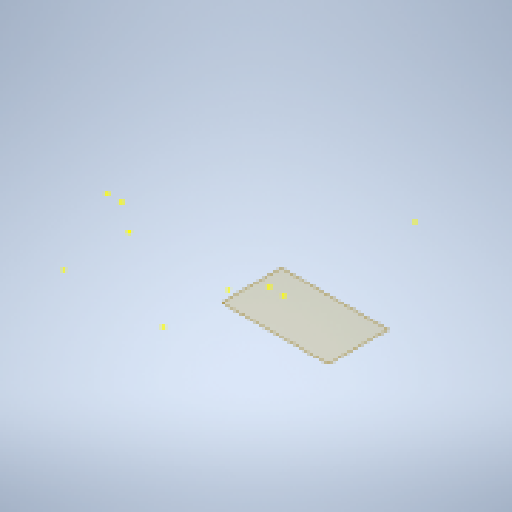
# Autodesk Inventor part: OCOTPUS_BOX_BACKING
Saved by Autodesk Inventor 2025.2 (Build 292293000, 293)
## iProperties
Created: 2026-03-26
Part Number: OCOTPUS_BOX_BACKING
Material: Generic
Document SubType Name: Sheet Metal
Designer: composite
Density: 1 g/cm^3
Sheet Metal Rule: Default_mm
Appearance: Default
Author: composite
Autodesk Inventor part; units mm, degrees
ref_plane "YZ Plane" through (0, 0, 0) normal (1, 0, 0) x (0, 1, 0)
ref_plane "XZ Plane" through (0, 0, 0) normal (0, 1, 0) x (-1, 0, 0)
ref_plane "XY Plane" through (0, 0, 0) normal (0, 0, 1) x (1, 0, 0)
ref_plane "Work Plane1" through (45.6354, 347.161, 237.8796) normal (0, 1, 0) x (-1, 0, 0)
sketch "Sketch1" plane through (45.6354, 347.161, 237.8796) normal (0, 1, 0) x (-1, 0, 0)
  circle A0 centre (74.35, -12.65) radius 2.75 projected
  circle A1 centre (49.35, -12.65) radius 2.75 projected
  circle A2 centre (355.85, -12.65) radius 2.75 projected
  circle A3 centre (330.85, -12.65) radius 2.75 projected
  circle A4 centre (278.85, 26.85) radius 2 projected
  circle A5 centre (278.85, 139.85) radius 2 projected
  circle A6 centre (105.85, 139.85) radius 2 projected
  circle A7 centre (105.85, 26.85) radius 2 projected
  line L0 (102.35, 141.35) -> (102.35, 25.35) projected
  circle A8 centre (105.85, 26.85) radius 3 projected
  circle A9 centre (278.85, 139.85) radius 3 projected
  circle A10 centre (117.35, 38.35) radius 1.75 projected
  circle A11 centre (267.35, 128.35) radius 1.75 projected
  circle A12 centre (267.35, 38.35) radius 1.75 projected
  circle A13 centre (117.35, 128.35) radius 1.75 projected
  arc A14 (280.35, 23.35) -> (282.35, 25.35) centre (280.35, 25.35) ccw projected
  line L1 (104.35, 23.35) -> (280.35, 23.35) projected
  arc A15 (102.35, 25.35) -> (104.35, 23.35) centre (104.35, 25.35) ccw projected
  line L2 (102.35, 141.35) -> (102.35, 25.35) projected
  arc A16 (104.35, 143.35) -> (102.35, 141.35) centre (104.35, 141.35) ccw projected
  line L3 (280.35, 143.35) -> (104.35, 143.35) projected
  arc A17 (282.35, 141.35) -> (280.35, 143.35) centre (280.35, 141.35) ccw projected
  line L4 (282.35, 25.35) -> (282.35, 141.35) projected
  circle A18 centre (105.85, 139.85) radius 3 projected
  circle A19 centre (278.85, 26.85) radius 3 projected
  line L5 (-3.9627, -32.65) -> (79.35, -32.65) projected
  line L6 (409.1627, -32.65) -> (325.85, -32.65) projected
  point P0 (45.6354, -237.8796)
sketch "Sketch2" plane through (45.6354, 347.161, 237.8796) normal (0, 1, 0) x (-1, 0, 0)
  arc A0 (104.35, 143.35) -> (102.35, 141.35) centre (104.35, 141.35) ccw
  line L0 (280.35, 143.35) -> (104.35, 143.35)
  arc A1 (282.35, 141.35) -> (280.35, 143.35) centre (280.35, 141.35) ccw
  circle A2 centre (278.85, 139.85) radius 2
  circle A3 centre (105.85, 139.85) radius 2
  circle A4 centre (105.85, 26.85) radius 2
  circle A5 centre (278.85, 26.85) radius 2
  line L1 (104.35, 23.35) -> (280.35, 23.35)
  circle A6 centre (330.85, -12.65) radius 2.75
  circle A7 centre (355.85, -12.65) radius 2.75
  circle A8 centre (49.35, -12.65) radius 2.75
  circle A9 centre (74.35, -12.65) radius 2.75
  line L2 (-3.9627, -32.65) -> (79.35, -32.65)
  line L3 (409.1627, -32.65) -> (325.85, -32.65)
  circle A10 centre (74.35, -12.65) radius 3.25
  circle A11 centre (49.35, -12.65) radius 3.25
  circle A12 centre (330.85, -12.65) radius 3.25
  circle A13 centre (355.85, -12.65) radius 3.25
  line L4 (79.35, -32.65) -> (115.85, 23.35)
  line L5 (115.85, 23.35) -> (268.85, 23.35)
  line L6 (268.85, 23.35) -> (325.85, -32.65)
  line L7 (370.85, -32.65) -> (370.85, 7.35)
  line L8 (370.85, 7.35) -> (282.35, 68.35)
  line L9 (282.35, 68.35) -> (282.35, 141.35)
  line L10 (34.35, -32.65) -> (34.35, 7.35)
  line L11 (34.35, 7.35) -> (102.35, 83.35)
  line L12 (102.35, 141.35) -> (102.35, 83.35)
  point P0 (45.6354, -237.8796)
  dimension "d0" = 0.5
  dimension "d1" = 0.5
  dimension "d2" = 0.5
  dimension "d3" = 0.5
  dimension "d4" = 45
  dimension "d5" = 45
  dimension "d6" = 60
  dimension "d7" = 75
  dimension "d8" = 10
  dimension "d9" = 10
  dimension "d10" = 40
  dimension "d11" = 40
  measures "d0" radial gap between concentric circles of A9 A10
  measures "d1" radial gap between concentric circles of A8 A11
  measures "d2" radial gap between concentric circles of A6 A12
  measures "d3" radial gap between concentric circles of A7 A13
  measures "d4" distance of L10.start L2.end
  measures "d5" distance of L7.start L3.end
  measures "d6" distance from line of L11.end L0
  measures "d7" distance from line of L0 L8.end
  measures "d8" horizontal distance of A4.centre L4.end
  measures "d9" horizontal distance of L5.end A5.centre
  measures "d10" distance of L10.start L10.end
  measures "d11" distance of L7.start L7.end
extrude "Plate1" add sketch "Sketch2" along normal blind 2 contours L0 A1 L9 L8 L7 L3 L6 L1 L4 L2 L10 L11 L12 A0
fillet "Corner Round1" radius 8 10 edges at (-56.7146, 348.161, 321.2296) (11.2854, 348.161, 245.2296) (11.2854, 348.161, 205.2296) (-33.7146, 348.161, 205.2296) (-70.2146, 348.161, 261.2296) (-223.2146, 348.161, 261.2296) (-280.2146, 348.161, 205.2296) (-325.2146, 348.161, 205.2296) (-325.2146, 348.161, 245.2296) (-236.7146, 348.161, 306.2296)
sketch "Sketch3" plane through (45.6354, 349.161, 237.8796) normal (0, 1, 0) x (1, 0, 0)
  circle A0 centre (-105.85, -26.85) radius 2 projected
  line L0 (-105.85, -26.85) -> (-278.85, -139.85) construction
  line L1 (-105.85, -139.85) -> (-278.85, -26.85) construction
  line L2 (-105.85, -139.85) -> (-105.85, -26.85)
  line L3 (-102.35, -141.35) -> (-102.35, -86.4065) projected
  line L4 (-105.85, -26.85) -> (-278.85, -26.85)
  circle A1 centre (-278.85, -139.85) radius 2 projected
  line L5 (-278.85, -26.85) -> (-278.85, -139.85)
  line L6 (-278.85, -139.85) -> (-105.85, -139.85)
  line L7 (-115.85, -129.85) -> (-115.85, -36.85)
  line L8 (-115.85, -36.85) -> (-268.85, -36.85)
  line L9 (-268.85, -129.85) -> (-105.85, -129.85)
  line L10 (-268.85, -36.85) -> (-268.85, -129.85)
  line L11 (-115.85, -42.9372) -> (-248.9112, -129.85)
  line L12 (-115.85, -123.7628) -> (-248.9112, -36.85)
  line L13 (-135.7888, -129.85) -> (-268.85, -42.9372)
  line L14 (-135.7888, -36.85) -> (-268.85, -123.7628)
  point P0 (-45.6354, 237.8796)
  point P1 (-105.85, -26.85)
  point P2 (-192.35, -73.7946)
  point P3 (-177.721, -83.35)
  point P4 (-192.35, -92.9054)
  point P5 (-206.979, -83.35)
  dimension "d15" = 10
  dimension "d16" = 10
  dimension "d17" = 10
  dimension "d18" = 10
  dimension "d23" = 8
  dimension "d24" = 8
  dimension "d25" = 8
  dimension "d26" = 8
  dimension "d27" = 3.5
  constraints: 28 end point, 9 point on line, 7 parallel, 2 perpendicular, 1 vertical
  measures "d15" distance between parallel lines of L2 L7
  measures "d16" distance between parallel lines of L4 L8
  measures "d17" distance between parallel lines of L6 L9
  measures "d18" distance between parallel lines of L5 L10
  measures "d23" distance between parallel lines of L1 L13
  measures "d24" distance between parallel lines of L1 L12
  measures "d25" distance between parallel lines of L0 L11
  measures "d26" distance between parallel lines of L14 L0
  measures "d27" distance from line of L9.end L3
extrude "Cut1" cut sketch "Sketch3" against normal blind 2 contours L12 L11 L7 | L9 L11 L13 | L12 L8 L14 | L14 L10 L13
fillet "Corner Round2" radius 8 12 edges at (-70.2146, 348.161, 361.6424) (-132.0856, 348.161, 321.2296) (-70.2146, 348.161, 280.8167) (-90.1534, 348.161, 274.7296) (-146.7146, 348.161, 311.6742) (-203.2759, 348.161, 274.7296) (-223.2146, 348.161, 280.8167) (-223.2146, 348.161, 361.6424) (-161.3436, 348.161, 321.2296) (-146.7146, 348.161, 330.7849) (-203.2759, 348.161, 367.7296) (-90.1534, 348.161, 367.7296)
equation "\"d4\" = d5"
equation "\"d9\" = d8"
equation "\"d11\" = d10"
equation "\"d16\" = d15"
equation "\"d17\" = d15"
equation "\"d18\" = d15"
equation "\"d24\" = d23"
equation "\"d25\" = d23"
equation "\"d26\" = d23"
equation "\"d28\" = Thickness"
equation "\"d13\" = Thickness"
equation "\"Thickness\" = 2"
body "Solid1"
